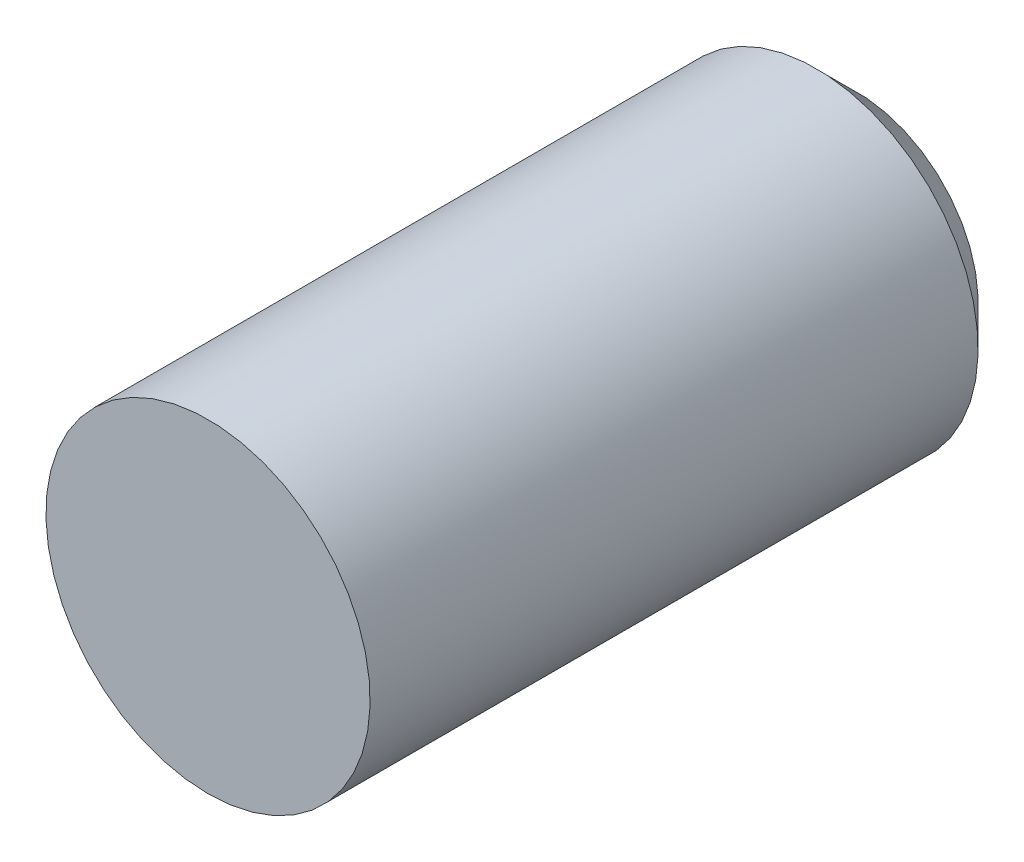
# Autodesk Inventor part: Dose_unten
Saved by Autodesk Inventor 2020 (Build 240168000, 168)
## iProperties
Created: 2020-03-21
Part Number: Dose_unten
Material: Generisch
Document SubType Name: Modeling
Designer: franz
Density: 1 g/cm^3
Appearance: Vorgabe
Author: franz
Autodesk Inventor part; units mm, degrees
ref_plane "YZ Plane" through (0, 0, 0) normal (1, 0, 0) x (0, 1, 0)
ref_plane "XZ Plane" through (0, 0, 0) normal (0, 1, 0) x (-1, 0, 0)
ref_plane "XY Plane" through (0, 0, 0) normal (0, 0, 1) x (1, 0, 0)
sketch "Skizze2" plane through (0, 0, 0) normal (1, 0, 0) x (0, 1, 0)
  line L0 (0, -33.6907) -> (0, 203.7987)
  line L1 (0, 0) -> (-30, 0)
  line L2 (-30, 0) -> (-40, 10)
  line L3 (-40, 10) -> (-40, 160)
  line L4 (-40, 160) -> (0, 160)
  dimension "d0" = 160
  dimension "d1" = 80
  dimension "d2" = 45
  dimension "d3" = 10
  constraints: 10 end point, 2 perpendicular, 2 vertical, 1 horizontal, 1 point on line
  measures "d0" distance between parallel lines of L1 L4
  measures "d1" diameter of L3 L0
  measures "d2" angle of L1 L2
  measures "d3" distance from line of L1 L2.end
revolve "Umdrehung1" add sketch "Skizze2" angle 360 about axis through (0, 0, -33.6907) along (0, 0, 1)
